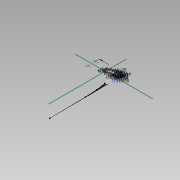
# Autodesk Inventor part: ShiftRail-34L-HLD
Saved by Autodesk Inventor 2021 (Build 250183000, 183)
## iProperties
Created: 2021-06-06
Part Number: ShiftRail-34L-HLD
Material: 一般
Document SubType Name: Modeling
Designer: kumagai
Density: 1 g/cm^3
Appearance: 既定
Author: kumagai
Autodesk Inventor part; units mm, degrees
ref_plane "YZ Plane" through (0, 0, 0) normal (1, 0, 0) x (0, 1, 0)
ref_plane "XZ Plane" through (0, 0, 0) normal (0, 1, 0) x (-1, 0, 0)
ref_plane "XY Plane" through (0, 0, 0) normal (0, 0, 1) x (1, 0, 0)
sketch "スケッチ1" plane through (0, 0, 0) normal (0, 1, 0) x (-1, 0, 0)
  line L0 (0, -129.227957) -> (0, 345.579773)
  line L1 (-289.551159, 0) -> (185.361867, 0)
  line L2 (-80.625, -23.75) -> (-79.742476, -23.75)
  arc A0 (-79.742476, -23.75) -> (-71.342986, -23.669821) centre (-79.742476, 416.25) ccw
  arc A1 (-71.342986, -23.669821) -> (-62.949618, -23.349191) centre (-75.542731, 196.29009) ccw
  arc A2 (-62.949618, -23.349191) -> (-54.58174, -22.62854) centre (-71.345026, 123.076996) ccw
  arc A3 (-54.58174, -22.62854) -> (-46.281535, -21.350923) centre (-67.154205, 86.650612) ccw
  arc A4 (-46.281535, -21.350923) -> (-38.122679, -19.366103) centre (-62.979671, 65.050305) ccw
  line L3 (-54.734409, 37.048713) -> (-59.227307, 52.306965)
  line L4 (-0.768566, -0.495589) -> (0, 0)
  arc A5 (-47.59082, -14.576281) -> (-40.071693, -12.747089) centre (-62.979671, 65.050305) ccw
  arc A6 (-55.370377, -15.773757) -> (-47.59082, -14.576281) centre (-67.154205, 86.650612) ccw
  arc A7 (-63.344584, -16.460504) -> (-55.370377, -15.773757) centre (-71.345026, 123.076996) ccw
  arc A8 (-71.474705, -16.771078) -> (-63.344584, -16.460504) centre (-75.542731, 196.29009) ccw
  arc A9 (-79.742476, -16.85) -> (-71.474705, -16.771078) centre (-79.742476, 416.25) ccw
  line L5 (-79.742476, -16.85) -> (-80.625, -16.85)
  arc A10 (-48.046224, -12.219884) -> (-40.749611, -10.444824) centre (-62.979671, 65.050305) ccw
  arc A11 (-55.644685, -13.389485) -> (-48.046224, -12.219884) centre (-67.154205, 86.650612) ccw
  arc A12 (-63.481963, -14.064439) -> (-55.644685, -13.389485) centre (-71.345026, 123.076996) ccw
  arc A13 (-71.52052, -14.371515) -> (-63.481963, -14.064439) centre (-75.542731, 196.29009) ccw
  arc A14 (-79.742476, -14.45) -> (-71.52052, -14.371515) centre (-79.742476, 416.25) ccw
  line L6 (-79.742476, -14.45) -> (-80.625, -14.45)
  arc A15 (-49.507311, -4.659777) -> (-42.924598, -3.058388) centre (-62.979671, 65.050305) ccw
  arc A16 (-56.524757, -5.739944) -> (-49.507311, -4.659777) centre (-67.154205, 86.650612) ccw
  arc A17 (-63.922722, -6.377065) -> (-56.524757, -5.739944) centre (-71.345026, 123.076996) ccw
  arc A18 (-71.667512, -6.672918) -> (-63.922722, -6.377065) centre (-75.542731, 196.29009) ccw
  arc A19 (-79.742476, -6.75) -> (-71.667512, -6.672918) centre (-79.742476, 416.25) ccw
  line L7 (-79.742476, -6.75) -> (-80.625, -6.75)
  arc A20 (-49.886814, -2.696113) -> (-43.489529, -1.139833) centre (-62.979671, 65.050305) ccw
  arc A21 (-56.753348, -3.75305) -> (-49.886814, -2.696113) centre (-67.154205, 86.650612) ccw
  arc A22 (-64.037205, -4.380344) -> (-56.753348, -3.75305) centre (-71.345026, 123.076996) ccw
  arc A23 (-71.705691, -4.673283) -> (-64.037205, -4.380344) centre (-75.542731, 196.29009) ccw
  arc A24 (-79.742476, -4.75) -> (-71.705691, -4.673283) centre (-79.742476, 416.25) ccw
  line L8 (-79.742476, -4.75) -> (-80.625, -4.75)
  arc A25 (-44.972249, -28.125565) -> (-36.173665, -25.985117) centre (-62.979671, 65.050305) ccw
  arc A26 (-53.793104, -29.483323) -> (-44.972249, -28.125565) centre (-67.154205, 86.650612) ccw
  arc A27 (-62.554652, -30.237877) -> (-53.793104, -29.483323) centre (-71.345026, 123.076996) ccw
  arc A28 (-71.211267, -30.568563) -> (-62.554652, -30.237877) centre (-75.542731, 196.29009) ccw
  arc A29 (-79.742476, -30.65) -> (-71.211267, -30.568563) centre (-79.742476, 416.25) ccw
  line L9 (-79.742476, -30.65) -> (-80.625, -30.65)
  arc A30 (-44.516845, -30.481962) -> (-35.495747, -28.287382) centre (-62.979671, 65.050305) ccw
  arc A31 (-53.518795, -31.867596) -> (-44.516845, -30.481962) centre (-67.154205, 86.650612) ccw
  arc A32 (-62.417273, -32.633942) -> (-53.518795, -31.867596) centre (-71.345026, 123.076996) ccw
  arc A33 (-71.165451, -32.968126) -> (-62.417273, -32.633942) centre (-75.542731, 196.29009) ccw
  arc A34 (-79.742476, -33.05) -> (-71.165451, -32.968126) centre (-79.742476, 416.25) ccw
  line L10 (-79.742476, -33.05) -> (-80.625, -33.05)
  arc A35 (-43.055758, -38.04207) -> (-33.32076, -35.673818) centre (-62.979671, 65.050305) ccw
  arc A36 (-52.638723, -39.517136) -> (-43.055758, -38.04207) centre (-67.154205, 86.650612) ccw
  arc A37 (-61.976514, -40.321317) -> (-52.638723, -39.517136) centre (-71.345026, 123.076996) ccw
  arc A38 (-71.01846, -40.666723) -> (-61.976514, -40.321317) centre (-75.542731, 196.29009) ccw
  arc A39 (-79.742476, -40.75) -> (-71.01846, -40.666723) centre (-79.742476, 416.25) ccw
  line L11 (-79.742476, -40.75) -> (-80.625, -40.75)
  arc A40 (-42.676255, -40.005734) -> (-32.755828, -37.592373) centre (-62.979671, 65.050305) ccw
  arc A41 (-52.410133, -41.50403) -> (-42.676255, -40.005734) centre (-67.154205, 86.650612) ccw
  arc A42 (-61.862031, -42.318038) -> (-52.410133, -41.50403) centre (-71.345026, 123.076996) ccw
  arc A43 (-70.980281, -42.666358) -> (-61.862031, -42.318038) centre (-75.542731, 196.29009) ccw
  arc A44 (-79.742476, -42.75) -> (-70.980281, -42.666358) centre (-79.742476, 416.25) ccw
  line L12 (-79.742476, -42.75) -> (-80.625, -42.75)
  line L13 (-79.742476, -42.75) -> (-79.742476, -4.75)
  line L14 (-80.625, -42.75) -> (-80.625, -4.75)
  line L15 (-32.755828, -37.592373) -> (-43.489529, -1.139833)
  line L16 (10.296597, -15.968096) -> (-10.296597, 15.968096)
  line L17 (-10.296597, 15.968096) -> (-11.065162, 15.472507)
  line L18 (-11.065162, 15.472507) -> (9.528031, -16.463685)
  line L19 (9.528031, -16.463685) -> (10.296597, -15.968096)
  line L20 (9.212744, -14.287244) -> (8.444178, -14.782833)
  line L21 (4.271347, -8.311552) -> (5.039913, -7.815963)
  line L22 (3.73929, -5.79894) -> (2.970724, -6.294529)
  line L23 (-4.507856, 5.303351) -> (-3.73929, 5.79894)
  line L24 (-5.039913, 7.815963) -> (-5.808479, 7.320374)
  line L25 (-9.98131, 13.791655) -> (-9.212744, 14.287244)
  point P0 (80.625, -23.75)
  point P1 (80.625, 23.75)
  point P2 (-80.625, 23.75)
  point P3 (-29.044432, -6.586083)
  point P4 (-31.154215, -1.843931)
  point P5 (-20.775665, -27.447499)
  point P6 (-52.696261, -6.75)
  point P7 (-52.696261, -16.85)
  point P8 (-52.696261, -14.45)
  point P9 (-52.696261, -33.05)
  point P10 (-52.696261, -30.65)
  point P11 (-52.696261, -40.75)
  dimension "d0" = 161.25
  dimension "d1" = 47.5
  dimension "d2" = 88
  dimension "d3" = 8.4
  dimension "d4" = 110
  dimension "d5" = 146.66667
  dimension "d6" = 220
  dimension "d7" = 440
  dimension "d11" = 8.4
  dimension "d12" = 8.4
  dimension "d17" = 8.4
  dimension "d18" = 8.4
  dimension "d19" = 38
  dimension "d21" = 2
  dimension "d22" = 18.6
  dimension "d23" = 2.4
  dimension "d27" = 421
  dimension "d28" = 201
  dimension "d29" = 127.66667
  dimension "d30" = 91
  dimension "d31" = 69
  dimension "d38" = 38
  dimension "d39" = 2
  dimension "d40" = 18.6
  dimension "d41" = 2.4
  constraints: 90 point on circle, 45 centre point, 39 end point, 5 tangent, 4 parallel, 4 symmetric about line, 1 horizontal, 1 line through centre, 1 point on line, 94 other
  measures "d0" distance of L2.start point (80.625, -23.75)
  measures "d1" distance of L2.start point (-80.625, 23.75)
  measures "d2" radius of A4
  measures "d4" radius of A3
  measures "d5" radius of A2
  measures "d6" radius of A1
  measures "d7" radius of A0
  measures "d19" distance between parallel lines of L8 L12
  measures "d21" distance between parallel lines of L12 L11
  measures "d22" distance between parallel lines of L6 L10
  measures "d23" distance between parallel lines of L9 L10
  measures "d27" radius of A24
  measures "d28" radius of A23
  measures "d29" radius of A22
  measures "d30" radius of A21
  measures "d31" radius of A20
  measures "d38" distance between parallel lines of L17 L19
  measures "d39" distance between parallel lines of L19 L20
  measures "d40" distance between parallel lines of L24 L21
  measures "d41" distance between parallel lines of L21 L22
sketch "スケッチ2" plane through (0, 0, 0) normal (0, 1, 0) x (-1, 0, 0)
  line L0 (-64.5, 0) -> (10.75, 0)
  line L1 (-80.625, -42.75) -> (-80.625, -4.75)
  line L2 (-80.625, -23.75) -> (-79.742476, -23.75)
  line L3 (-80.625, -30.65) -> (-68.625, -30.65)
  line L4 (-68.625, -30.65) -> (-68.625, -16.85)
  line L5 (-68.625, -16.85) -> (-80.625, -16.85)
  line L6 (-80.625, -16.85) -> (-80.625, -30.65)
  point P0 (0, 0)
  point P1 (-80.625, -16.85)
  dimension "d48" = 13.8
  dimension "d49" = 12
  constraints: 8 end point, 2 parallel, 1 horizontal, 1 perpendicular, 1 point on line, 1 other
  measures "d48" distance between parallel lines of L5 L3
  measures "d49" distance between parallel lines of L1 L4
extrude "押し出し1" add sketch "スケッチ1" against normal blind 2 contours L13 A9 A8 A7 A6 A5 L15 A4 A3 A2 A1 A0 | A0 A1 A2 A3 A4 L15 A25 A26 A27 A28 A29 L13 | A29 A28 A27 A26 A25 L15 A30 A31 A32 A33 A34 L13 | L13 A14 A13 A12 A11 A10 L15 A5 A6 A7 A8 A9 | A34 A33 A32 A31 A30 L15 A35 A36 A37 A38 A39 L13 | L13 A19 A18 A17 A16 A15 L15 A10 A11 A12 A13 A14 | A39 A38 A37 A36 A35 L15 A40 A41 A42 A43 A44 L13 | L13 A24 A23 A22 A21 A20 L15 A15 A16 A17 A18 A19
extrude "押し出し2" add sketch "スケッチ1" along normal blind 3.2 and the other way blind 5.2 contours A29 A28 A27 A26 A25 L15 A30 A31 A32 A33 A34 L13 | L13 A14 A13 A12 A11 A10 L15 A5 A6 A7 A8 A9 | A39 A38 A37 A36 A35 L15 A40 A41 A42 A43 A44 L13 | L13 A24 A23 A22 A21 A20 L15 A15 A16 A17 A18 A19
mirror "ミラー1" about plane through (43.489529, 0, -1.139833) normal (-0.9592774, 0, 0.2824658) of "押し出し1", "押し出し2"
extrude "押し出し3" add sketch "スケッチ1" against normal blind 2 contours L18 L4 L0 | L0 L16 L22 L18 | L4 L18 L1 | L1 L18 L23 L16 | L22 L16 L21 L18 | L23 L18 L24 L16 | L21 L16 L20 L18 | L24 L18 L25 L16 | L20 L16 L19 L18 | L25 L18 L17 L16 | L14 L5 L13 L2 | L2 L13 L9 L14 | L9 L13 L10 L14 | L14 L6 L13 L5 | L10 L13 L11 L14 | L14 L7 L13 L6 | L11 L13 L12 L14 | L14 L8 L13 L7
extrude "押し出し4" add sketch "スケッチ1" along normal blind 3.2 and the other way blind 5.2 contours L22 L16 L21 L18 | L23 L18 L24 L16 | L20 L16 L19 L18 | L25 L18 L17 L16 | L9 L13 L10 L14 | L14 L6 L13 L5 | L11 L13 L12 L14 | L14 L8 L13 L7
extrude "押し出し5" cut sketch "スケッチ2" against normal blind 2
chamfer "面取り1" distance 0.8 angle 45 96 edges at (2.804, 0, -21.7827) (10.8295, 0, -26.302) (19.3915, 0, -30.4962) (28.5491, 0, -34.1441) (38.16, 0, -36.9741) (47.8332, 0, -38.8711) (57.3019, 0, -39.9861) (66.4958, 0, -40.5372) (75.3803, 0, -40.7292) (80.1837, 0, -40.75) (-4.7668, 0, -17.1293) (-8.8285, 0, -14.535) (33.2553, 0, 0.5488) (26.7352, 0, 3.7481) (20.1253, 0, 7.4743) (13.3851, 0, 11.6197) (9.597, 0, 14.0394) (39.698, 0, -2.024) (46.1968, 0, -3.9376) (53.0057, 0, -5.2669) (60.2192, 0, -6.1115) (67.7937, 0, -6.562) (75.7048, 0, -6.7307) (80.1837, 0, -6.75) (19.3915, -2, -30.4962) (10.8295, -2, -26.302) (2.804, -2, -21.7827) (-4.7668, -2, -17.1293) (-8.8285, -2, -14.535) (38.16, -2, -36.9741) (28.5491, -2, -34.1441) (47.8332, -2, -38.8711) (57.3019, -2, -39.9861) (66.4958, -2, -40.5372) (75.3803, -2, -40.7292) (80.1837, -2, -40.75) (26.7352, -2, 3.7481) (33.2553, -2, 0.5488) (39.698, -2, -2.024) (46.1968, -2, -3.9376) (53.0057, -2, -5.2669) (60.2192, -2, -6.1115) (67.7937, -2, -6.562) (75.7048, -2, -6.7307) (80.1837, -2, -6.75) (20.1253, -2, 7.4743) (13.3851, -2, 11.6197) (9.597, -2, 14.0394) (30.1156, -2, -6.482) (23.1331, -2, -3.0574) (16.2025, -2, 0.8485) (9.2742, -2, 5.1089) (5.4242, -2, 7.5682) (37.1731, -2, -9.2983) (44.3767, -2, -11.4194) (51.8343, -2, -12.8772) (59.5585, -2, -13.7831) (67.4998, -2, -14.2563) (75.6313, -2, -14.4304) (80.1837, -2, -14.45) (22.5312, -2, -23.4655) (31.074, -2, -26.8699) (39.9801, -2, -29.4923) (49.0046, -2, -31.2607) (57.9625, -2, -32.3145) (66.7898, -2, -32.8428) (75.4538, -2, -33.0295) (80.1837, -2, -33.05) (14.4317, -2, -19.4965) (6.7267, -2, -15.1568) (-0.6559, -2, -10.6185) (-4.6556, -2, -8.0638) (22.5312, 0, -23.4655) (14.4317, 0, -19.4965) (6.7267, 0, -15.1568) (-0.6559, 0, -10.6185) (-4.6556, 0, -8.0638) (31.074, 0, -26.8699) (39.9801, 0, -29.4923) (49.0046, 0, -31.2607) (57.9625, 0, -32.3145) (66.7898, 0, -32.8428) (75.4538, 0, -33.0295) (80.1837, 0, -33.05) (16.2025, 0, 0.8485) (23.1331, 0, -3.0574) (30.1156, 0, -6.482) (37.1731, 0, -9.2983) (44.3767, 0, -11.4194) (51.8343, 0, -12.8772) (59.5585, 0, -13.7831) (67.4998, 0, -14.2563) (75.6313, 0, -14.4304) (80.1837, 0, -14.45) (9.2742, 0, 5.1089) (5.4242, 0, 7.5682)
equation "\"d0\" = Length"
equation "\"d1\" = Shift"
equation "\"d3\" = SLength"
equation "\"d11\" = SLength"
equation "\"d12\" = SLength"
equation "\"d18\" = SLength"
equation "\"d19\" = RailWidth"
equation "\"d21\" = OuterWall"
equation "\"d22\" = InsideWidth"
equation "\"d23\" = InnerWall"
equation "\"d38\" = RailWidth"
equation "\"d39\" = OuterWall"
equation "\"d40\" = InsideWidth"
equation "\"d41\" = InnerWall"
equation "\"d32\" = RailHeight - 2 * RailDepth"
equation "\"d34\" = RailDepth"
equation "\"d42\" = RailHeight - 2 * RailDepth"
equation "\"d44\" = RailDepth"
equation "\"d45\" = RailHeight - RailDepth"
equation "\"Length\" = 161.25"
equation "\"Shift\" = 47.5"
equation "\"MinRadius\" = 88"
equation "\"CLength\" = 42"
equation "\"SD\" = 0"
equation "\"SLength\" = 8.4"
equation "\"RailWidth\" = 38"
equation "\"OuterWall\" = 2"
equation "\"InsideWidth\" = 18.6"
equation "\"InnerWall\" = 2.4"
equation "\"RailHeight\" = 8.4"
equation "\"RailDepth\" = 3.2"
